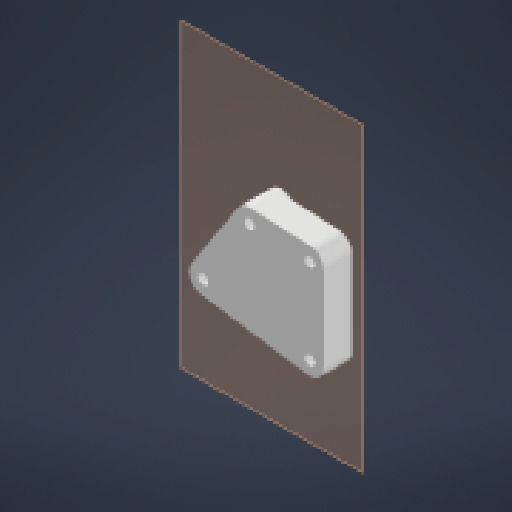
# Autodesk Inventor part: Intake
Saved by Autodesk Inventor 2026.1 (Build 301233000, 233)
## iProperties
Created: 2025-09-11
Part Number: Intake
Material: Generic
Document SubType Name: Modeling
Designer: Teddy
Density: 1 g/cm^3
Appearance: Default
Author: Teddy
Autodesk Inventor part; units mm, degrees
ref_plane "YZ Plane" through (0, 0, 0) normal (1, 0, 0) x (0, 1, 0)
ref_plane "XZ Plane" through (0, 0, 0) normal (0, 1, 0) x (-1, 0, 0)
ref_plane "Work Plane1" through (0, 0, 0) normal (0, 0, 1) x (1, 0, 0)
sketch "Sketch1" plane through (0, 0, 0) normal (0, 0, 1) x (1, 0, 0)
  circle A0 centre (-53.3761, -75.183) radius 2.286 projected
  circle A1 centre (-32.6369, -43.2221) radius 2.286 projected
  line L0 (-53.3761, -75.183) -> (-32.6369, -43.2221) construction
  line L1 (-48.0493, -78.6395) -> (-27.3101, -46.6786)
  line L2 (-37.9638, -39.7656) -> (-58.7029, -71.7265)
  arc A2 (-58.7029, -71.7265) -> (-48.0493, -78.6395) centre (-53.3761, -75.183) ccw
  arc A3 (-27.3101, -46.6786) -> (-37.9638, -39.7656) centre (-32.6369, -43.2221) ccw
  line L3 (-55.5272, -90.1636) -> (-13.3531, -25.1695) projected
  point P0 (0, 0)
  point P1 (-43.0065, -59.2025)
  constraints: 8 end point, 4 point on circle, 4 tangent, 2 centre point, 1 midpoint, 1 parallel, 1 point on line
ref_plane "Work Plane2" through (-11.9062, -368.3, 1.8415) normal (0, 0, 1) x (1, 0, 0)
extrude "Extrusion1" add sketch "Sketch1" along normal up to surface (1.8415 mm away)
sketch "Sketch2" plane through (-58.7029, -71.7265, 1.8415) normal (0, 0, 1) x (0.8388686, -0.544334, 0)
  circle A0 centre (29.7355, 51.8109) radius 2.1844 projected
  circle A1 centre (50.4747, 19.85) radius 2.1844 projected
  line L0 (0, 0) -> (0, 38.1) projected
  arc A2 (0, 0) -> (12.7, 0) centre (6.35, 0) ccw projected
  line L1 (12.7, 38.1) -> (12.7, 0) projected
  arc A3 (12.7, 38.1) -> (0, 38.1) centre (6.35, 38.1) ccw projected
  circle A4 centre (6.35, 0) radius 2.286 projected
  circle A5 centre (6.35, 38.1) radius 2.286 projected
  arc A6 (35.0623, 55.2674) -> (26.5238, 57.2888) centre (29.7355, 51.8109) ccw
  arc A7 (53.0798, 14.059) -> (55.8015, 23.3065) centre (50.4747, 19.85) ccw
  line L2 (26.5238, 57.2888) -> (3.1383, 43.5779)
  line L3 (35.0623, 55.2674) -> (55.8015, 23.3065)
  line L4 (53.0798, 14.059) -> (8.9552, -5.791)
  point P0 (10.2009, 92.1231)
  dimension "d2" = 12.7
  dimension "d3" = 12.7
  constraints: 6 end point, 6 point on circle, 6 tangent, 2 centre point, 2 coincident
  measures "d2" diameter of A6
  measures "d3" diameter of A7
extrude "Extrusion2" add sketch "Sketch2" along normal blind 12.7
body "Solid1"
